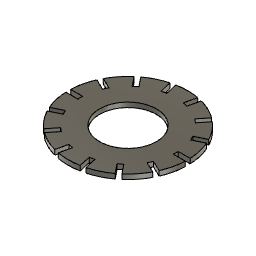
Hringur_Litill (Autodesk Fusion 360 design; units mm, degrees)
Autodesk Fusion 360 part; units mm, degrees
sketch "Sketch1" plane through (0, 0, 0) normal (0, 0, 1) x (1, 0, 0)
  circle A0 centre (0, 0) radius 23.75
  line L0 (49.96, 2) -> (39.96, 2)
  line L1 (39.96, 2) -> (39.96, -2)
  line L2 (39.96, -2) -> (49.96, -2)
  line L3 (44.1446, 23.4788) -> (35.1349, 19.1399)
  line L4 (36.8705, 15.536) -> (45.8802, 19.8749)
  line L5 (35.1349, 19.1399) -> (36.8705, 15.536)
  line L6 (29.5859, 40.3073) -> (23.351, 32.489)
  line L7 (26.4783, 29.995) -> (32.7132, 37.8133)
  line L8 (23.351, 32.489) -> (26.4783, 29.995)
  line L9 (9.1673, 49.1524) -> (6.9421, 39.4031)
  line L10 (10.8418, 38.5131) -> (13.067, 48.2623)
  line L11 (6.9421, 39.4031) -> (10.8418, 38.5131)
  line L12 (-13.067, 48.2623) -> (-10.8418, 38.5131)
  line L13 (-6.9421, 39.4031) -> (-9.1673, 49.1524)
  line L14 (-10.8418, 38.5131) -> (-6.9421, 39.4031)
  line L15 (-32.7132, 37.8133) -> (-26.4783, 29.995)
  line L16 (-23.351, 32.489) -> (-29.5859, 40.3073)
  line L17 (-26.4783, 29.995) -> (-23.351, 32.489)
  line L18 (-45.8802, 19.8749) -> (-36.8705, 15.536)
  line L19 (-35.1349, 19.1399) -> (-44.1446, 23.4788)
  line L20 (-36.8705, 15.536) -> (-35.1349, 19.1399)
  line L21 (-49.96, -2) -> (-39.96, -2)
  line L22 (-39.96, 2) -> (-49.96, 2)
  line L23 (-39.96, -2) -> (-39.96, 2)
  line L24 (-44.1446, -23.4788) -> (-35.1349, -19.1399)
  line L25 (-36.8705, -15.536) -> (-45.8802, -19.8749)
  line L26 (-35.1349, -19.1399) -> (-36.8705, -15.536)
  line L27 (-29.5859, -40.3073) -> (-23.351, -32.489)
  line L28 (-26.4783, -29.995) -> (-32.7132, -37.8133)
  line L29 (-23.351, -32.489) -> (-26.4783, -29.995)
  line L30 (-9.1673, -49.1524) -> (-6.9421, -39.4031)
  line L31 (-10.8418, -38.5131) -> (-13.067, -48.2623)
  line L32 (-6.9421, -39.4031) -> (-10.8418, -38.5131)
  line L33 (13.067, -48.2623) -> (10.8418, -38.5131)
  line L34 (6.9421, -39.4031) -> (9.1673, -49.1524)
  line L35 (10.8418, -38.5131) -> (6.9421, -39.4031)
  line L36 (32.7132, -37.8133) -> (26.4783, -29.995)
  line L37 (23.351, -32.489) -> (29.5859, -40.3073)
  line L38 (26.4783, -29.995) -> (23.351, -32.489)
  line L39 (45.8802, -19.8749) -> (36.8705, -15.536)
  line L40 (35.1349, -19.1399) -> (44.1446, -23.4788)
  line L41 (36.8705, -15.536) -> (35.1349, -19.1399)
  arc A1 (49.96, 2) -> (45.8802, 19.8749) centre (0, 0) ccw
  arc A2 (44.1446, 23.4788) -> (32.7132, 37.8133) centre (0, 0) ccw
  arc A3 (29.5859, 40.3073) -> (13.067, 48.2623) centre (0, 0) ccw
  arc A4 (9.1673, 49.1524) -> (-9.1673, 49.1524) centre (0, 0) ccw
  arc A5 (-13.067, 48.2623) -> (-29.5859, 40.3073) centre (0, 0) ccw
  arc A6 (-32.7132, 37.8133) -> (-44.1446, 23.4788) centre (0, 0) ccw
  arc A7 (-45.8802, 19.8749) -> (-49.96, 2) centre (0, 0) ccw
  arc A8 (-49.96, -2) -> (-45.8802, -19.8749) centre (0, 0) ccw
  arc A9 (-44.1446, -23.4788) -> (-32.7132, -37.8133) centre (0, 0) ccw
  arc A10 (-29.5859, -40.3073) -> (-13.067, -48.2623) centre (0, 0) ccw
  arc A11 (-9.1673, -49.1524) -> (9.1673, -49.1524) centre (0, 0) ccw
  arc A12 (13.067, -48.2623) -> (29.5859, -40.3073) centre (0, 0) ccw
  arc A13 (32.7132, -37.8133) -> (44.1446, -23.4788) centre (0, 0) ccw
  arc A14 (45.8802, -19.8749) -> (49.96, -2) centre (0, 0) ccw
  dimension "d1" = 100
  dimension "d6" = 47.5
  dimension "d7" = 10
  dimension "d8" = 10
  dimension "d9" = 4
  dimension "d11" = 360
  constraint coincident A0.centre A1.centre
  constraint horizontal L0
  constraint perpendicular L0 L1
  constraint perpendicular L1 L2
  constraint concentric A1 A2
  constraint concentric A2 A3
  constraint concentric A3 A4
  constraint concentric A4 A5
  constraint concentric A5 A6
  constraint concentric A6 A7
  constraint concentric A7 A8
  constraint concentric A8 A9
  constraint concentric A9 A10
  constraint concentric A10 A11
  constraint concentric A11 A12
  constraint concentric A12 A13
  constraint concentric A13 A14
  measures "d1" diameter of A1
  measures "d6" diameter of A0
  measures "d7" distance of L0.start L0.end
  measures "d8" distance of L1.end L2.end
  measures "d9" distance of L0.end L1.end
extrude "Extrude1" add sketch "Sketch1" along normal blind 4
equation "d1 = D_o"
equation "D_o = 100 mm"
equation "D_i = 47.5 mm"
equation "þykkt = 4 mm"
equation "offset = 10 mm"
equation "d6 = D_i"
equation "d7 = offset"
equation "d8 = offset"
equation "d9 = þykkt"
equation "d12 = þykkt"
